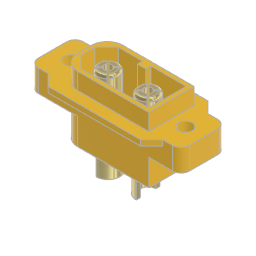
XT60E-M_panel (Autodesk Fusion 360 design; units mm, degrees)
Autodesk Fusion 360 part; units mm, degrees
sketch "Sketch1" plane through (0, 0, 0) normal (0, 1, 0) x (1, 0, 0)
  line L0 (0, 0) -> (0, -4.05) construction
  circle A0 centre (-3.6, 0) radius 2.125
  circle A1 centre (3.6, 0) radius 2.125
  line L1 (13.575, -4.05) -> (-13.575, -4.05)
  line L2 (-13.575, -4.05) -> (-13.575, 4.05)
  line L3 (-13.575, 4.05) -> (13.575, 4.05)
  line L4 (13.575, 4.05) -> (13.575, -4.05)
  line L5 (13.575, -4.05) -> (-13.575, 4.05) construction
  line L6 (-13.575, -4.05) -> (13.575, 4.05) construction
  line L7 (7.8, -4.05) -> (-7.8, -4.05)
  line L8 (-7.8, -4.05) -> (-7.8, 4.05)
  line L9 (-7.8, 4.05) -> (7.8, 4.05)
  line L10 (7.8, 4.05) -> (7.8, -4.05)
  line L11 (7.8, -4.05) -> (-7.8, 4.05) construction
  line L12 (-7.8, -4.05) -> (7.8, 4.05) construction
  line L13 (-10.3, -4.05) -> (-8.3, -6.05)
  line L14 (-8.3, -6.05) -> (8.3, -6.05)
  line L15 (8.3, -6.05) -> (10.3, -4.05)
  circle A2 centre (-10.3, 0) radius 1.25
  line L16 (0, 0) -> (-13.575, 0) construction
  circle A3 centre (10.3, 0) radius 1.25
  line L17 (-10.3, 4.05) -> (-8.3, 6.05)
  line L18 (-8.3, 6.05) -> (8.3, 6.05)
  line L19 (8.3, 6.05) -> (10.3, 4.05)
  arc A4 (-7.8, -1.25) -> (-5, -4.05) centre (-5, -1.25) ccw
  arc A5 (-5, 4.05) -> (-7.8, 1.25) centre (-5, 1.25) ccw
  line L20 (-6.1598, -4.05) -> (-10.2098, 0) construction
  line L21 (-0.75, -3.35) -> (0.75, -3.35)
  line L22 (0.75, -3.35) -> (0.75, -2.45)
  line L23 (0.75, -2.45) -> (-0.75, -2.45)
  line L24 (-0.75, -2.45) -> (-0.75, -3.35)
  line L25 (-5.1, -3.35) -> (7.1, -3.35)
  line L26 (7.1, -3.35) -> (7.1, 3.35)
  line L27 (7.1, 3.35) -> (-5.1, 3.35)
  line L28 (-5.1, 3.35) -> (-7.2, 1.25)
  line L29 (-7.2, 1.25) -> (-7.2, -1.25)
  line L30 (-7.2, -1.25) -> (-5.1, -3.35)
  circle A6 centre (-3.6, 0) radius 1.875
  circle A7 centre (-3.6, 0) radius 0.75
  line L31 (-5.0113, -1.2345) -> (-4.2113, -0.4345)
  line L32 (-4.8345, -1.4113) -> (-4.0345, -0.6113)
  line L33 (-3.6, 0) -> (-4.9258, -1.3258) construction
  line L34 (-2.1887, -1.2345) -> (-2.9887, -0.4345)
  line L35 (-2.3655, -1.4113) -> (-3.1655, -0.6113)
  line L36 (-2.3655, 1.4113) -> (-3.1655, 0.6113)
  line L37 (-2.1887, 1.2345) -> (-2.9887, 0.4345)
  line L38 (-5.0113, 1.2345) -> (-4.2113, 0.4345)
  line L39 (-4.8345, 1.4113) -> (-4.0345, 0.6113)
  circle A8 centre (3.6, 0) radius 1.875
  line L40 (4.8345, -1.4113) -> (4.0345, -0.6113)
  line L41 (5.0113, -1.2345) -> (4.2113, -0.4345)
  circle A9 centre (3.6, 0) radius 0.75
  line L42 (2.3655, -1.4113) -> (3.1655, -0.6113)
  line L43 (2.1887, -1.2345) -> (2.9887, -0.4345)
  line L44 (2.1887, 1.2345) -> (2.9887, 0.4345)
  line L45 (2.3655, 1.4113) -> (3.1655, 0.6113)
  line L46 (4.8345, 1.4113) -> (4.0345, 0.6113)
  line L47 (5.0113, 1.2345) -> (4.2113, 0.4345)
  line L48 (-7.85, 1.4145) -> (-10.3, 2.829)
  line L49 (-10.3, 2.829) -> (-12.75, 1.4145)
  line L50 (-12.75, 1.4145) -> (-12.75, -1.4145)
  line L51 (-12.75, -1.4145) -> (-10.3, -2.829)
  line L52 (-10.3, -2.829) -> (-7.85, -1.4145)
  line L53 (-7.85, -1.4145) -> (-7.85, 1.4145)
  line L54 (12.75, -1.4145) -> (10.3, -2.829)
  line L55 (10.3, -2.829) -> (7.85, -1.4145)
  line L56 (7.85, -1.4145) -> (7.85, 1.4145)
  line L57 (7.85, 1.4145) -> (10.3, 2.829)
  line L58 (10.3, 2.829) -> (12.75, 1.4145)
  line L59 (12.75, 1.4145) -> (12.75, -1.4145)
  point P0 (-7.2, 0)
  point P1 (-10.3, 0)
  dimension "d1" = 4.25
  dimension "d2" = 7.2
  dimension "d3" = 27.15
  dimension "d4" = 8.1
  dimension "d5" = 15.6
  dimension "d6" = 2
  dimension "d7" = 45
  dimension "d8" = 45
  dimension "d9" = 20.6
  dimension "d10" = 2.5
  dimension "d15" = 45
  dimension "d16" = 15.5986
  dimension "d19" = 1.5
  dimension "d20" = 0.9
  dimension "d21" = 0.7
  dimension "d22" = 0.7
  dimension "d23" = 0.7
  dimension "d24" = 0.6
  dimension "d25" = 2.5
  dimension "d26" = 135
  dimension "d28" = 2.5
  dimension "d40" = 3.75
  dimension "d41" = 1.5
  dimension "d42" = 0.25
  dimension "d44" = 45
  dimension "d46" = 360
  dimension "d47" = 4.9
  constraint coincident L0.start L16.start
  constraint vertical L0
  constraint symmetric L0 A0 A1
  constraint horizontal L1
  constraint perpendicular L1 L2
  constraint parallel L1 L3
  constraint parallel L2 L4
  constraint coincident L5 L0.start
  constraint coincident L6 L0.start
  constraint horizontal L7
  constraint perpendicular L7 L8
  constraint parallel L7 L9
  constraint parallel L8 L10
  constraint coincident L1 L7.start
  constraint coincident L11 L0.start
  constraint coincident L12 L0.start
  constraint midpoint L0.end L1
  constraint coincident L1 L13.start
  constraint parallel L1 L14
  constraint coincident L1 L15.end
  constraint midpoint L2 L16.end
  constraint coincident P1 L16
  constraint coincident A0.centre L16
  constraint symmetric L0 A2 A3
  constraint vertical L13.start P1
  constraint vertical L15.end A3.centre
  constraint symmetric L13.start L16 L17.start
  constraint symmetric L13.end L16 L17.end
  constraint symmetric L14.end L16 L18.end
  constraint symmetric L15.end L16 L19.end
  constraint coincident L8 A4.start
  constraint coincident L1 A4.end
  constraint tangent L7 A4
  constraint tangent L8 A4
  constraint symmetric L16 A4.end A5.start
  constraint symmetric L16 A4.start A5.end
  constraint symmetric L16 A4 A5
  constraint coincident L1 L20.start
  constraint coincident L16 L20.end
  constraint tangent A4 L20
  constraint horizontal L21
  constraint vertical L22
  constraint horizontal L23
  constraint vertical L24
  constraint horizontal L25
  constraint perpendicular L25 L26
  constraint perpendicular L26 L27
  constraint parallel L26 L29
  constraint perpendicular L28 L30
  constraint midpoint L29 P0
  constraint coincident L16 P0
  constraint collinear L21 L25
  constraint concentric A0 A6
  constraint concentric A6 A7
  constraint coincident A6 L31.start
  constraint coincident A7 L31.end
  constraint coincident A6 L32.start
  constraint coincident A7 L32.end
  constraint parallel L31 L32
  constraint coincident A0.centre A6.centre
  constraint coincident A6 L33.end
  constraint parallel L31 L33
  constraint symmetric L31 L32 L33
  constraint symmetric L0 A6 A8
  constraint symmetric L0 A7 A9
  constraint symmetric L0 L31.start L41.start
  constraint symmetric L0 L31.end L41.end
  constraint symmetric L0 L32.start L40.start
  constraint symmetric L0 L32.end L40.end
  constraint symmetric L0 L34.start L43.start
  constraint symmetric L0 L34.end L43.end
  constraint symmetric L0 L35.start L42.start
  constraint symmetric L0 L35.end L42.end
  constraint symmetric L0 L36.start L45.start
  constraint symmetric L0 L36.end L45.end
  constraint symmetric L0 L37.start L44.start
  constraint symmetric L0 L37.end L44.end
  constraint symmetric L0 L38.start L47.start
  constraint symmetric L0 L38.end L47.end
  constraint symmetric L0 L39.start L46.start
  constraint symmetric L0 L39.end L46.end
  constraint coincident P1 A2.centre
  constraint perpendicular L16 L53
  constraint symmetric L0 L48.start L56.end
  constraint symmetric L0 L48.end L57.end
  constraint symmetric L0 L49.end L58.end
  constraint symmetric L0 L50.end L54.start
  constraint symmetric L0 L51.end L54.end
  constraint symmetric L0 L52.end L55.end
  measures "d1" diameter of A0
  measures "d2" distance of A0.centre A1.centre
  measures "d3" distance of L2.end L3.end
  measures "d4" distance of L1.end L2.end
  measures "d5" distance of L8.end L9.end
  measures "d6" distance of L7 L14
  measures "d7" angle of L1 L13
  measures "d8" angle of L1 L15
  measures "d9" distance of P1 A3.centre
  measures "d10" diameter of A2
  measures "d15" angle of L1 L20
  measures "d16" distance of L9.end L20
  measures "d19" distance of L22.end L23.end
  measures "d20" distance of L21.end L22.end
  measures "d21" distance of L7 L25
  measures "d22" distance of L10 L26
  measures "d23" distance of L9 L27
  measures "d24" distance of A5.end L29
  measures "d25" distance of L28.end L29.end
  measures "d26" angle of L29 L30
  measures "d28" distance of A5.centre A4.centre
  measures "d40" diameter of A6
  measures "d41" diameter of A7
  measures "d42" distance of L31 L32
  measures "d44" angle of L16 L33
  measures "d47" distance of L50 L53
extrude "Extrude1" add sketch "Sketch1" along normal blind 4 contours L1 L3 L4 L10 | L1 L3 L7 L8 L9 L10 A4 A5 | L1 L7 L8 A4 | L1 L2 L3 L8 | L3 L8 L9 A5 | L48 L49 L50 L51 L52 L53 | L54 L55 L56 L57 L58 L59 makes body 1
extrude "Extrude2" add sketch "Sketch1" along normal blind 1 contours L1 L7 L13 L14 L15 | L3 L9 L17 L18 L19 bodies 1
extrude "Extrude3" add sketch "Sketch1" against normal blind 3 contours L1 L3 L7 L8 L9 L10 A4 A5 bodies 1
extrude "Extrude4" add sketch "Sketch1" along normal blind 8.75 contours L1 L3 L7 L8 L9 L10 A4 A5 bodies 1
extrude "Extrude5" add sketch "Sketch1" along normal blind 2.05 from surface at 5.7 contours L21 L22 L23 L24 L25 | L22 L23 L24 L25 L26 L27 L28 L29 L30 bodies 1
extrude "Extrude6" add sketch "Sketch1" along normal up to surface (5.7 mm away) and the other way up to surface (3 mm away) contours L21 L22 L23 L24 L25 bodies 1
extrude "Extrude7" cut sketch "Sketch1" against normal blind 2 from surface at 4 contours L48 L49 L50 L51 L52 L53 | L54 L55 L56 L57 L58 L59 bodies 1
fillet "Fillet1" radius 1.5 4 edges at (13.575, 2, 4.05) (13.575, 2, -4.05) (-13.575, 2, 4.05) (-13.575, 2, -4.05) on bodies 1
extrude "Extrude1'" add sketch "Sketch1" along normal up to surface (2 mm away) from surface at 2 separate body contours L48 L49 L50 L51 L52 L53 | L54 L55 L56 L57 L58 L59 makes body 2 at (-9.275, 2, -1.7754) makes body 3 at (9.275, 2, -1.7754) in component "nuts"
chamfer "Chamfer1" distance 0.2 angle 45 4 faces at (9.275, 4, -1.7754) (9.275, 2, -1.7754) (-9.275, 4, -1.7754) (-9.275, 2, -1.7754) on bodies 2 3 in component "nuts"
extrude "Extrude1''" add sketch "Sketch1" along normal blind -0.5 and the other way blind -8 from surface at 5.7 separate body contours A0 | A1 | A6 A7 L34 L37 | A6 A7 L36 L37 | A6 A7 L34 L35 | A6 A7 L36 L39 | A7 | A6 A7 L32 L35 | A6 A7 L38 L39 | A6 A7 L31 L32 | A6 A7 L31 L38 | A8 L41 A9 L47 | A8 A9 L46 L47 | A8 L40 L41 A9 | A8 A9 L45 L46 | A9 | A8 L40 A9 L42 | A8 A9 L44 L45 | A8 A9 L42 L43 | A8 A9 L43 L44 makes body 4 at (-1.4776, 8.0333, 0.1059) makes body 5 at (5.7224, 8.0333, 0.1059) in component "pins"
extrude "Extrude2'" add sketch "Sketch1" against normal blind 8 from surface at 5.7 contours A6 A7 L34 L37 | A6 A7 L36 L39 | A6 A7 L32 L35 | A6 A7 L31 L38 | A8 L41 A9 L47 | A8 A9 L45 L46 | A8 L40 A9 L42 | A8 A9 L43 L44 bodies 4 5 in component "pins"
fillet "Fillet1'" radius 0.5 8 edges at (-3.6, -2.3, 1.875) (-1.725, -2.3, 0) (-5.475, -2.3, 0) (-3.6, -2.3, -1.875) (3.6, -2.3, -1.875) (1.725, -2.3, 0) (3.6, -2.3, 1.875) (5.475, -2.3, 0) on bodies 4 5 in component "pins"
sketch "Sketch1 (2)" plane through (0, 13.7, 0) normal (0, 1, 0) x (-1, 0, 0) in component "pins"
  circle A0 centre (-3.6, 0) radius 2.125
  line L0 (-3.6, 2.125) -> (-3.6, -2.125)
  circle A1 centre (-3.6, 0) radius 1.375
  circle A2 centre (3.6, 0) radius 2.125
  line L1 (3.6, 2.125) -> (3.6, -2.125)
  circle A3 centre (3.6, 0) radius 1.375
  dimension "d67" = -0.75
  dimension "d74" = -0.75
  constraint coincident A0 L0.start
  constraint vertical L0
  constraint coincident A0.centre L0
  constraint coincident A0 L0.end
  constraint coincident A2 L1.start
  constraint coincident A2 L1.end
  constraint vertical L1
  constraint coincident A2.centre L1
extrude "Extrude3'" cut sketch "Sketch1 (2)" against normal blind 3 contours A0 L0 A1 | A2 L1 A3 picked at (-4.739, -1.4832) picked at (5.4631, -0.166) bodies 4 5 in component "pins"
extrude "Extrude4'" cut sketch "Sketch1 (2)" against normal blind 6.5 contours L0 A1 | L0 A1 | L1 A3 | L1 A3 bodies 4 5 in component "pins"
fillet "Fillet2" radius 1.35 2 faces at (-3.6048, 7.2, 0.3617) (4.0129, 7.2, 0.4083) on bodies 4 5 in component "pins"
copy_body "CutPasteBodies1" bodies 1 removing the originals makes body 6 in component "housing"
component "housing" placed x (1, 0, 0) y (0, 0, -1) z (0, 1, 0) at (0, 2.6437, 2.6837)
component "nuts" placed x (1, 0, 0) y (0, 0, -1) z (0, 1, 0) at (0, 2.6437, 2.6837)
component "pins" placed x (1, 0, 0) y (0, 0, -1) z (0, 1, 0) at (0, 2.6437, 2.6837)
equation "d34 = 7.75 mm - 5.7 mm"
